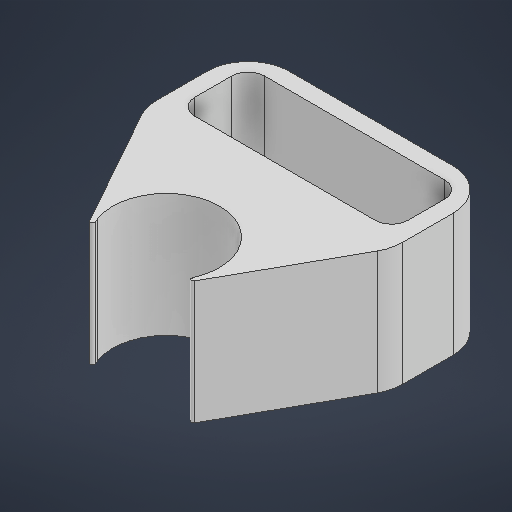
# Autodesk Inventor part: Turret_Holder_2_test_pt2
Saved by Autodesk Inventor 2026.2 (Build 302298000, 298)
## iProperties
Created: 2025-12-30
Part Number: Turret_Holder_2_test_pt2
Material: Generic
Document SubType Name: Modeling
Designer: Cobble
Density: 1 g/cm^3
Appearance: Default
Author: Cobble
Autodesk Inventor part; units mm, degrees
ref_plane "YZ Plane" through (0, 0, 0) normal (1, 0, 0) x (0, 1, 0)
ref_plane "XZ Plane" through (0, 0, 0) normal (0, 1, 0) x (-1, 0, 0)
ref_plane "XY Plane" through (0, 0, 0) normal (0, 0, 1) x (1, 0, 0)
sketch "Sketch1" plane through (0, 0, 0) normal (0, 0, 1) x (1, 0, 0)
  line L0 (-5.2, 1.7) -> (5.2, 1.7)
  line L1 (5.2, 1.7) -> (5.2, -1.7)
  line L2 (5.2, -1.7) -> (-5.2, -1.7)
  line L3 (-5.2, -1.7) -> (-5.2, 1.7)
  line L4 (-5.2, 1.7) -> (5.2, -1.7) construction
  line L5 (5.2, 1.7) -> (-5.2, -1.7) construction
  line L6 (0, 0) -> (0, -7.5)
  circle A0 centre (0, -7.5) radius 2.6
  line L7 (-6, 2.5) -> (6, 2.5)
  line L8 (6, 2.5) -> (6, -2.5)
  line L9 (6, -2.5) -> (-6, -2.5)
  line L10 (-6, -2.5) -> (-6, 2.5)
  line L11 (-6, 2.5) -> (6, -2.5) construction
  line L12 (6, 2.5) -> (-6, -2.5) construction
  circle A1 centre (0, -7.5) radius 2.8
  line L13 (-6, -2.5) -> (-2.4445, -8.8654)
  line L14 (6, -2.5) -> (2.4445, -8.8654)
  line L15 (0, -7.5) -> (2.1964, -10.1176)
  line L16 (0, -7.5) -> (3.417, -7.5) construction
  line L17 (0, -7.5) -> (-2.5132, -10.4951)
  line L18 (0, -7.5) -> (3.9099, -7.5) construction
  line L19 (2.4445, -8.8654) -> (1.9255, -9.7947)
  line L20 (-2.4445, -8.8654) -> (-1.9255, -9.7947)
  line L21 (-1.9255, -9.7947) -> (-2.4397, -8.3988)
  line L22 (1.9255, -9.7947) -> (2.4397, -8.3988)
  point P0 (-2.2345, -8.8294)
  point P1 (2.2345, -8.8294)
  point P2 (-2.5783, -7.8348)
  point P3 (2.5783, -7.8348)
  dimension "d0" = 10.4
  dimension "d1" = 3.4
  dimension "d2" = 7.5
  dimension "d3" = 5.2
  dimension "d4" = 12
  dimension "d5" = 5
  dimension "d9" = 5.6
  dimension "d10" = 50
  dimension "d11" = 130
  constraints: 46 end point, 8 point on circle, 6 tangent, 4 horizontal, 4 midpoint, 4 parallel, 2 centre point, 2 coincident, 2 equal length, 2 perpendicular, 2 point on line, 1 vertical
  measures "d0" distance of L1.end L2.end
  measures "d1" distance of L0.end L1.end
  measures "d2" distance of L6.start L6.end
  measures "d3" diameter of A0
  measures "d4" distance of L8.end L9.end
  measures "d5" distance of L7.end L8.end
  measures "d9" diameter of A1
  measures "d10" angle of L15 L16
  measures "d11" angle of L17 L18
extrude "Extrusion1" add sketch "Sketch1" along normal blind 6 contours L9 L10 L7 L8 | L9 L14 A1 L6 | L6 A1 L13 L9 | A1 L22 A0 L6 | L6 A0 L21 A1 | A1 L21 L20 | L19 L22 A1
fillet "Fillet1" radius 2 4 edges at (-6, 2.5, 3) (6, 2.5, 3) (-6, -2.5, 3) (6, -2.5, 3)
fillet "Fillet2" radius 0.1 2 edges at (-1.9255, -9.7947, 3) (1.9255, -9.7947, 3)
fillet "Fillet3" radius 0.8 4 edges at (5.2, -1.7, 3) (5.2, 1.7, 3) (-5.2, -1.7, 3) (-5.2, 1.7, 3)
body "Solid1"
